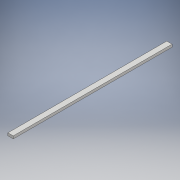
# Autodesk Inventor part: Pieza4
Saved by Autodesk Inventor 2017 (Build 210142000, 142)
## iProperties
Part Number: Pieza4
Material: Genérico
Document SubType Name: Modeling
Designer: diego
Density: 1 g/cm^3
Appearance: Valor por defecto
Author: diego
Autodesk Inventor part; units mm, degrees
ref_plane "YZ Plane" through (0, 0, 0) normal (1, 0, 0) x (0, 1, 0)
ref_plane "XZ Plane" through (0, 0, 0) normal (0, 1, 0) x (-1, 0, 0)
ref_plane "XY Plane" through (0, 0, 0) normal (0, 0, 1) x (1, 0, 0)
sketch "Boceto1" plane through (0, 0, 0) normal (0, 0, 1) x (1, 0, 0)
  line L0 (0, 0) -> (0, 600)
  line L1 (0, 600) -> (20, 600)
  line L2 (20, 600) -> (20, 0)
  line L3 (20, 0) -> (0, 0)
  dimension "d0" = 600
  dimension "d2" = 20
  dimension "d3" = 600
  constraints: 8 end point, 1 horizontal, 1 perpendicular, 1 vertical
  measures "d0" distance of L0.start L0.end
  measures "d2" distance of L0.end L1.end
  measures "d3" distance of L1.end L2.end
extrude "Extrusión1" add sketch "Boceto1" along normal blind 10
